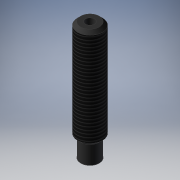
# Autodesk Inventor part: C-AC0806M_b
Saved by Autodesk Inventor 2019 (Build 230136000, 136)
## iProperties
Created: 2023-10-14
Part Number: C-AC0806M_b
Material: Generic
Catalog Web Link: www.cadenas.de
Description: C-AC____, C-AC____-N_body-C-VALUE Shock Absorbers - Double-stage Type
Vendor: MISUMI
Document SubType Name: Modeling
Designer: psAdmin
Manufacturer: MISUMI
Mass: 1.62071 g
Surface Area: 11.6688 cm^2
Volume: 1.62071 cm^3
Density: 1 g/cm^3
Appearance: PSOLRGB-175-175-175
Category: PARTsolutions
Company: MISUMI
Title: C-AC0806M
Author: Cadenas PARTsolutions
Comments: C-VALUE Shock Absorbers - Double-stage Type
PSOL_IDENT_0: {$CADENAS_DATA/23d-libs/misumi/metric/29_springs/c_ac____/c_ac_____body.prj},184 {VTYP=3D},{NB=C-AC0
PSOL_IDENT_1: 806M_b},{LINA=C-AC0806M},{NN=C-AC____, C-AC____-N_body},{DATE=28.09.2022 00:58:29},{GEOMDATE=19.05.2
PSOL_IDENT_2: 022 00:37:57},{VERSION=},{LINEID=180},{WBVAR=TS,V},{WBNUMERIC=}  {NB=C-AC0806M_b},{LINA=C-AC0806M},{
PSOL_IDENT_3: KT=DUMMY},{PN=C-AC0806M},{TYPE=C-AC0806M},{TS=Cap},{TSALG= 'Cap','Cap','No Cap','No Cap' },{NO=0806}
PSOL_IDENT_4: ,{V=M},{M=M8x1.0},{M3D=8},{PITCH=1.00},{S=6},{L=50.0},{L1=32.0},{L2=6.0},{T=4.0},{TT=6.0},{DD=6.6},{
PSOL_IDENT_5: DD1=2.9},{B=11.0},{LW=With},{LW1=15.0},{LW2=17.0},{NUT1=7.000},{NUT2=23.000},{C3D=6.000},{L3=20},{C=
PSOL_IDENT_6: 0.2},{C1=1.00}
NB: C-AC0806M_b
NN: C-AC____, C-AC____-N_body
NT: C-VALUE Shock Absorbers - Double-stage Type
NBSYN: $PN._b
LINA: C-AC0806M
CATALOG: Misumi
PN: C-AC0806M
TS: Cap
NO: 0806
V: M
M: M8x1.0
S: 6
L: 50
L1: 32
L2: 6
T: 4
TT: 6
DD: 6.6
DD1: 2.9
B: 11
LW: With
SUPPLIER: MISUMI
ARTICLENO: C-AC0806M_b
BOMINFO: C-AC0806M
CREATOR: CADENAS GmbH
Autodesk Inventor part; units mm, degrees
sketch "Sketch_1" plane through (0, 0, 0) normal (0, 0, 1) x (1, 0, 0)
  line L0 (0, -38) -> (0, 38)
  line L1 (0, 32) -> (3, 32)
  line L2 (3, 32) -> (4, 31)
  line L3 (4, 31) -> (4, 1)
  line L4 (4, 1) -> (3, 0)
  line L5 (3, 0) -> (3, -5.8)
  line L6 (3, -5.8) -> (2.8, -6)
  line L7 (2.8, -6) -> (0, -6)
  line L8 (0, -6) -> (0, 32)
  constraints: 18 end point
revolve "Revolution1" add sketch "Sketch_1" angle 360 about axis through (0, -38, 0) along (0, -1, 0)
thread "Thread1" size "M8x1" class "6g" standard "ISO Metric profile" full length
sketch "Sketch2" plane through (0, 32, 0) normal (0, 1, 0) x (1, 0, 0)
  point P0 (0, 0)
hole "Hole1" at (0, 32, 0) direction (0, -1, 0) diameter 2.9 depth 20 tip angle 118
ref_plane "to_cap_XY" through (0, 38, 0) normal (0, -1, 0) x (1, 0, 0)
ref_plane "to_cap_YZ" through (0, 38, 0) normal (1, 0, 0) x (0, 0, 1)
ref_plane "to_cap_ZX" through (0, 38, 0) normal (0, 0, 1) x (0, -1, 0)
ref_plane "to_nut1_XY" through (0, 7, 0) normal (0, -1, 0) x (1, 0, 0)
ref_plane "to_nut1_YZ" through (0, 7, 0) normal (1, 0, 0) x (0, 0, 1)
ref_plane "to_nut1_ZX" through (0, 7, 0) normal (0, 0, 1) x (0, -1, 0)
ref_plane "to_nut2_XY" through (0, 23, 0) normal (0, -1, 0) x (1, 0, 0)
ref_plane "to_nut2_YZ" through (0, 23, 0) normal (1, 0, 0) x (0, 0, 1)
ref_plane "to_nut2_ZX" through (0, 23, 0) normal (0, 0, 1) x (0, -1, 0)
ref_plane "to_rod_XY" through (0, 32, 0) normal (0, 1, 0) x (1, 0, 0)
ref_plane "to_rod_YZ" through (0, 32, 0) normal (1, 0, 0) x (0, 0, -1)
ref_plane "to_rod_ZX" through (0, 32, 0) normal (0, 0, -1) x (0, 1, 0)
ref_plane "to_washers_1_XY" through (0, 15, 0) normal (0, 1, 0) x (1, 0, 0)
ref_plane "to_washers_1_YZ" through (0, 15, 0) normal (1, 0, 0) x (0, 0, -1)
ref_plane "to_washers_1_ZX" through (0, 15, 0) normal (0, 0, -1) x (0, 1, 0)
ref_plane "to_washers_2_XY" through (0, 17, 0) normal (0, -1, 0) x (1, 0, 0)
ref_plane "to_washers_2_YZ" through (0, 17, 0) normal (1, 0, 0) x (0, 0, 1)
ref_plane "to_washers_2_ZX" through (0, 17, 0) normal (0, 0, 1) x (0, -1, 0)
body "Solid1"
